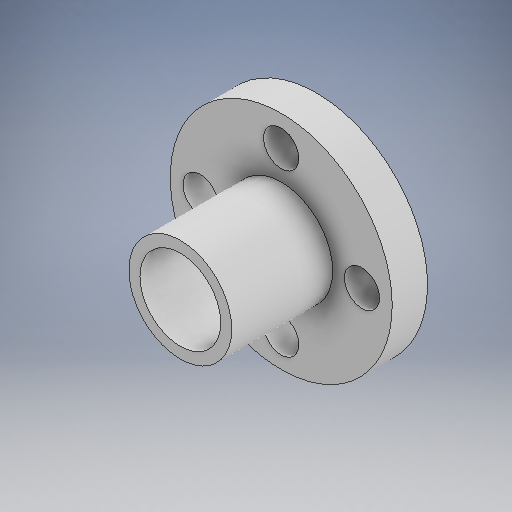
# Autodesk Inventor part: Porca_T8
Saved by Autodesk Inventor 2025.2 (Build 292293000, 293)
## iProperties
Created: 2025-04-06
Part Number: Porca_T8
Material: Generic
Document SubType Name: Modeling
Designer: Tiago
Density: 1 g/cm^3
Appearance: Default
Author: Tiago
Autodesk Inventor part; units mm, degrees
ref_plane "YZ Plane" through (0, 0, 0) normal (1, 0, 0) x (0, 1, 0)
ref_plane "XZ Plane" through (0, 0, 0) normal (0, 1, 0) x (-1, 0, 0)
sketch "Sketch1" plane through (0, 0, 0) normal (0, 0, 1) x (1, 0, 0)
  circle A0 centre (0, 0) radius 5.1
  circle A1 centre (0, 0) radius 4
  dimension "d0" = 10.2
  dimension "d1" = 8
  constraints: 2 centre point, 2 coincident
  measures "d0" diameter of A0
  measures "d1" diameter of A1
extrude "Extrusion1" add sketch "Sketch1" along normal blind 15
ref_plane "Work Plane1" through (0, 0, 1.5) normal (0, 0, 1) x (1, 0, 0)
sketch "Sketch2" plane through (0, 0, 1.5) normal (0, 0, 1) x (1, 0, 0)
  circle A0 centre (0, 0) radius 4 projected
  circle A1 centre (0, 0) radius 5.1 projected
  circle A2 centre (0, 0) radius 11
  circle A3 centre (0, 0) radius 8 construction
  circle A4 centre (0, -8) radius 1.75
  circle A5 centre (8, 0) radius 1.75
  circle A6 centre (0, 8) radius 1.75
  circle A7 centre (-8, 0) radius 1.75
  dimension "d6" = 16
  dimension "d5" = 22
  dimension "furos" = 3.5
  dimension "d10" = 360
  constraints: 5 centre point, 2 coincident, 1 vertical alignment, 11 other
  measures "d5" diameter of A2
  measures "furos" diameter of A4
extrude "Extrusion2" add sketch "Sketch2" along normal blind 3.5 contours A2
sketch "Sketch3" plane through (0, 0, 0) normal (1, 0, 0) x (0, 1, 0)
  line L0 (11, 5) -> (11, 1.5) projected
  line L1 (11, 1.5) -> (9.75, 1.5) projected
  line L2 (9.75, 1.5) -> (9.75, 5) projected
  line L3 (9.75, 5) -> (11, 5) projected
  line L4 (-11, 1.5) -> (-11, 5) projected
  line L5 (-11, 5) -> (-9.75, 5) projected
  line L6 (-9.75, 5) -> (-9.75, 1.5) projected
  line L7 (-9.75, 1.5) -> (-11, 1.5) projected
  line L8 (-4, 15) -> (-4, 0) projected
  line L9 (-4, 0) -> (-5.1, 0) projected
  line L10 (-5.1, 0) -> (-5.1, 1.5) projected
  line L11 (-5.1, 1.5) -> (-6.25, 1.5) projected
  line L12 (-6.25, 1.5) -> (-6.25, 5) projected
  line L13 (-6.25, 5) -> (-5.1, 5) projected
  line L14 (-5.1, 5) -> (-5.1, 15) projected
  line L15 (-5.1, 15) -> (-4, 15) projected
  line L16 (4, 0) -> (4, 15) projected
  line L17 (4, 15) -> (5.1, 15) projected
  line L18 (5.1, 15) -> (5.1, 5) projected
  line L19 (5.1, 5) -> (6.25, 5) projected
  line L20 (6.25, 5) -> (6.25, 1.5) projected
  line L21 (6.25, 1.5) -> (5.1, 1.5) projected
  line L22 (5.1, 1.5) -> (5.1, 0) projected
  line L23 (5.1, 0) -> (4, 0) projected
  point P0 (0, 0)
body "Solid1"
